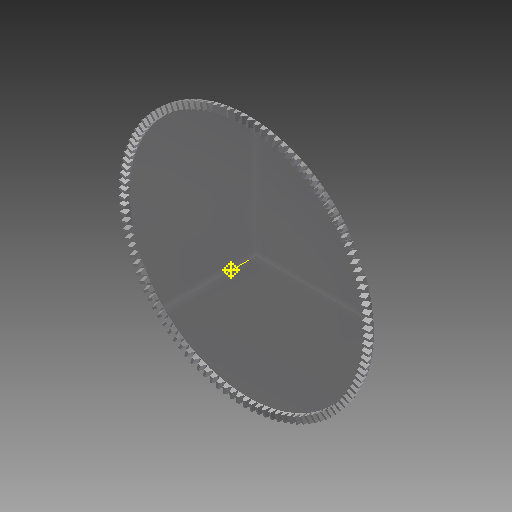
# Autodesk Inventor part: Bevel Gear1
Saved by Autodesk Inventor 2017 (Build 210142000, 142)
## iProperties
Created: 2017-01-10
Part Number: Bevel Gear1
Material: Steel, Mild
Document SubType Name: Modeling
Designer: David Kopala
Categories: <?xml version="1.0" encoding="UTF-16"?> <MemberInstance><Categories><FamilyTemplate><FamilyTemplateParameter ValueType="xs:double" Id="1" ObjectReferenceKey="da_z" ObjectType="kUserParameterObject"/><FamilyTemplateParameter ValueType="xs:double" Id="2" ObjectReferenceKey="da_b" ObjectType="kUserParameterObject"/><FamilyTemplateParameter ValueType="xs:double" Id="3" ObjectReferenceKey="da_beta" ObjectType="kUserParameterObject"/><FamilyTemplateParameter ValueType="xs:double" Id="4" ObjectReferenceKey="da_dae" ObjectType="kUserParameterObject"/><FamilyTemplateParameter ValueType="xs:double" Id="5" ObjectReferenceKey="da_ve" ObjectType="kUserParameterObject"/><FamilyTemplateParameter ValueType="xs:double" Id="6" ObjectReferenceKey="da_omega" ObjectType="kUserParameterObject"/><FamilyTemplateParameter ValueType="xs:string" Id="7" ObjectReferenceKey="EAIAABAAAAAAHwAAAAAAAIAAAAAAAAAA" ObjectType="83914240" SubObjectId="SurfaceGeometry"/></FamilyTemplate><ParamToTemplateMap><ParamToTemplate CategoryParameter="//CategoryParameter[@InternalName='046C89C9-8512-4d59-83FE-43B91F4F132A']" TemplateParameter="1"/><ParamToTemplate CategoryParameter="//CategoryParameter[@InternalName='2552DF32-E462-4b46-AEBF-C6C7768E72AC']" TemplateParameter="2"/><ParamToTemplate CategoryParameter="//CategoryParameter[@InternalName='C9EE641D-15FC-4fae-A226-E94C4372FDD7']" TemplateParameter="3"/><ParamToTemplate><ParamToTemplate CategoryParameter="//CategoryParameter[@InternalName='00B6519A-459B-49c7-AD84-2E56D39A5744']" ConstantValue="0.000000"/></ParamToTemplate><ParamToTemplate><ParamToTemplate CategoryParameter="//CategoryParameter[@InternalName='04B31F0E-C7A6-4894-AA32-9629BEFACF47']" ConstantValue="1.000000"/></ParamToTemplate><ParamToTemplate><ParamToTemplate CategoryParameter="//CategoryParameter[@InternalName='43CBEC2E-7847-49e7-A936-2F7889FCB2D9']" ConstantValue="0.200000"/></ParamToTemplate><ParamToTemplate><ParamToTemplate CategoryParameter="//CategoryParameter[@InternalName='B1EFC894-105D-4ebd-86BF-FA20ED196853']" ConstantValue="0.300000"/></ParamToTemplate><ParamToTemplate><ParamToTemplate CategoryParameter="//CategoryParameter[@InternalName='51175063-3D10-4879-93E8-6246FE8B403D']" ConstantValue="2061532430.657340"/></ParamToTemplate><ParamToTemplate><ParamToTemplate CategoryParameter="//CategoryParameter[@InternalName='A3A52E27-4454-46a9-B0BD-C932399B70AF']" ConstantValue="0.300000"/></ParamToTemplate><ParamToTemplate CategoryParameter="//CategoryParameter[@InternalName='2A200944-5A8C-41ca-B96E-8520D2E510F1']" TemplateParameter="4"/><ParamToTemplate><ParamToTemplate CategoryParameter="//CategoryParameter[@InternalName='1A637F62-92C8-44bc-B81F-10802510B579']" ConstantValue="27.761106"/></ParamToTemplate><ParamToTemplate CategoryParameter="//CategoryParameter[@InternalName='B52DD4BE-6863-48fb-BF58-89EF6F9EC65C']" TemplateParameter="5"/><ParamToTemplate><ParamToTemplate CategoryParameter="//CategoryParameter[@InternalName='3956BFF2-84D2-457d-93C2-9B0613DEBA67']" ConstantValue="1.567608"/></ParamToTemplate><ParamToTemplate CategoryParameter="//CategoryParameter[@InternalName='739CFA02-461B-4bf8-8049-181FCAD8B28F']" TemplateParameter="6"/><ParamToTemplate><ParamToTemplate CategoryParameter="//CategoryParameter[@InternalName='A27E999F-E2CE-4481-8A2A-EBF499C4C3C5']" ConstantValue="0.000000"/></ParamToTemplate><ParamToTemplate><ParamToTemplate CategoryParameter="//CategoryParameter[@InternalName='9E1B4470-B2D3-4ff1-B813-535BB4CDF51A']" ConstantValue="3523220.976809"/></ParamToTemplate><ParamToTemplate><ParamToTemplate CategoryParameter="//CategoryParameter[@InternalName='F8452263-BFF6-458c-9FB1-07C4B99E95CD']" ConstantValue="11397033.805607"/></ParamToTemplate><ParamToTemplate><ParamToTemplate CategoryParameter="//CategoryParameter[@InternalName='3E3BB259-FD49-497f-8171-6EBC954A3479']" ConstantValue="2.000000"/></ParamToTemplate><ParamToTemplate CategoryParameter="//CategoryParameter[@InternalName='27C3BAF2-7550-4e4b-AE2C-0DB134B7D9B7']" TemplateParameter="7"/></ParamToTemplateMap><Category DisplayName="Gear" InternalName="DC85795E-93AB-48d5-8EEE-5A27447B64BD" Mnemonic="Gear"><CategoryParameter DisplayName="z" InternalName="046C89C9-8512-4d59-83FE-43B91F4F132A" Mnemonic="z"/><CategoryParameter DisplayName="b" InternalName="2552DF32-E462-4b46-AEBF-C6C7768E72AC" Mnemonic="b"/><CategoryParameter DisplayName="||b|" InternalName="C9EE641D-15FC-4fae-A226-E94C4372FDD7" Mnemonic="beta"/><CategoryParameter DisplayName="x" InternalName="00B6519A-459B-49c7-AD84-2E56D39A5744" Mnemonic="x"/><CategoryParameter DisplayName="a*" InternalName="04B31F0E-C7A6-4894-AA32-9629BEFACF47" Mnemonic="a"/><CategoryParameter DisplayName="c*" InternalName="43CBEC2E-7847-49e7-A936-2F7889FCB2D9" Mnemonic="c"/><CategoryParameter DisplayName="r|.f|*" InternalName="B1EFC894-105D-4ebd-86BF-FA20ED196853" Mnemonic="rf"/><CategoryParameter DisplayName="E" InternalName="51175063-3D10-4879-93E8-6246FE8B403D" Mnemonic="E"/><CategoryParameter DisplayName="||m|" InternalName="A3A52E27-4454-46a9-B0BD-C932399B70AF" Mnemonic="mi"/><Category DisplayName="BevelGear" InternalName="0C98F69A-0C2B-4791-B2FE-7691BB227E77" Mnemonic="BevelGear"><CategoryParameter DisplayName="d|.ae|" InternalName="2A200944-5A8C-41ca-B96E-8520D2E510F1" Mnemonic="dae"/><CategoryParameter DisplayName="d|.ai|" InternalName="1A637F62-92C8-44bc-B81F-10802510B579" Mnemonic="dai"/><CategoryParameter DisplayName="A|.e|" InternalName="B52DD4BE-6863-48fb-BF58-89EF6F9EC65C" Mnemonic="ve"/><CategoryParameter DisplayName="A|.i|" InternalName="3956BFF2-84D2-457d-93C2-9B0613DEBA67" Mnemonic="vi"/><CategoryParameter DisplayName="||S|" InternalName="739CFA02-461B-4bf8-8049-181FCAD8B28F" Mnemonic="omega"/><CategoryParameter DisplayName="x|.t|" InternalName="A27E999F-E2CE-4481-8A2A-EBF499C4C3C5" Mnemonic="xt"/><CategoryParameter DisplayName="||s||.Flim|" InternalName="9E1B4470-B2D3-4ff1-B813-535BB4CDF51A" Mnemonic="sFlim"/><CategoryParameter DisplayName="||s||.Hlim|" InternalName="F8452263-BFF6-458c-9FB1-07C4B99E95CD" Mnemonic="sHlim"/><CategoryParameter DisplayName="type" InternalName="3E3BB259-FD49-497f-8171-6EBC954A3479" Mnemonic="type"/><CategoryParameter DisplayName="PitchDiameter" InternalName="27C3BAF2-7550-4e4b-AE2C-0DB134B7D9B7" Mnemonic="IDS_PITCHDIAM"/></Category></Category></Categories></MemberInstance>
Mass: 60.9118 g
Surface Area: 34.3074 cm^2
Volume: 7.7496 cm^3
Density: 7.86 g/cm^3
Appearance: Steel
CustomPartVersion: 1
Author: David Kopala
Autodesk Inventor part; units mm, degrees
ref_plane "XZ Plane" through (0, 0, 0) normal (0, 1, 0) x (-1, 0, 0)
ref_plane "Mesh Plane2" through (0, 0, 0) normal (0.9996269, 0.0273148, 0) x (0, 0, 1)
sketch "Teeth Body Sketch" plane through (0, 0, 0) normal (1, 0, 0) x (0, 1, 0)
  line L0 (0, 0) -> (145.6558, -22.0724) construction
  line L1 (145.6558, -22.0724) -> (146.3785, -16.5313)
  line L2 (146.3785, -16.5313) -> (0, 0) construction
  line L3 (146.05, -19.05) -> (0, 0) construction
  line L4 (138.1202, -20.9305) -> (138.8055, -15.6761)
  line L5 (145.6558, -22.0724) -> (138.1202, -20.9305)
  line L6 (146.3785, -16.5313) -> (138.8055, -15.6761)
  line L7 (0, -26.4874) -> (0, 4.4146) projected
  line L8 (0, -19.05) -> (146.3785, -19.05) construction
  dimension "d0" = 292.1
  dimension "d1" = 291.3116
  dimension "d2" = 292.757
  dimension "d3" = 7.62
  dimension "d4" = 16.5313
  constraints: 16 end point, 4 point on line, 3 perpendicular, 2 collinear, 1 horizontal alignment, 1 vertical alignment
  measures "d0" diameter of L3.start L7
  measures "d1" diameter of L0.end L7
  measures "d2" diameter of L1.end L7
  measures "d3" distance between parallel lines of L1 L4
  measures "d4" vertical distance of L1.end L0.start
revolve "Teeth Body" add sketch "Teeth Body Sketch" angle 360 about axis through (0, 0, 0) along (0, 0, 1)
ref_plane "Tooth Plane" through (0, 146.05, -19.05) normal (0, -0.9916004, 0.1293392) x (1, 0, 0)
sketch "Start Sketch" plane through (0, 146.05, -19.05) normal (0, -0.9916004, 0.1293392) x (1, 0, 0)
  line L0 (0, -1379.3559) -> (0, 234.8142) projected
  arc A0 (-0.7258, -3.7185) -> (-3.4846, 4.2111) centre (-367.6879, -126.9464) ccw
  arc A1 (3.4846, 4.2111) -> (0.7258, -3.7185) centre (367.6879, -126.9464) ccw
  line L1 (-0.7258, -3.7185) -> (0.7258, -3.7185)
  arc A2 (3.4846, 4.2111) -> (-3.4846, 4.2111) centre (0, -1129.2015) ccw
  dimension "d7" = 387.0999
  dimension "d8" = 367.6879
  dimension "d9" = 1002.255
  dimension "d57" = 1133.4179
  dimension "d58" = 1125.4829
  constraints: 6 point on circle, 3 centre point, 3 symmetric about line, 2 end point, 1 coincident, 1 perpendicular, 1 other
  measures "d7" radius of A0
  measures "d8" horizontal distance of point (0, -1129.201) A0.centre
  measures "d9" vertical distance of point (0, -1129.201) A0.centre
  measures "d57" radius of A2
  measures "d58" distance from line of A2.centre L1
sketch "End Sketch" plane through (0, 138.217, -18.0283) normal (0, -0.9916004, 0.1293392) x (1, 0, 0)
  line L0 (0, -1306.2352) -> (0, 223.7109) projected
  arc A0 (-0.6876, -2.3936) -> (-3.3012, 5.1186) centre (-348.3356, -119.1357) ccw
  arc A1 (3.3012, 5.1186) -> (0.6876, -2.3936) centre (348.3356, -119.1357) ccw
  line L1 (-0.6876, -2.3936) -> (0.6876, -2.3936)
  arc A2 (3.3012, 5.1186) -> (-3.3012, 5.1186) centre (0, -1068.6394) ccw
  dimension "d12" = 366.7258
  dimension "d15" = 348.3356
  dimension "d16" = 949.5037
  dimension "d59" = 1073.7631
  dimension "d60" = 1066.2458
  constraints: 6 point on circle, 3 centre point, 3 symmetric about line, 2 end point, 1 coincident, 1 other
  measures "d12" radius of A0
  measures "d15" horizontal distance of A0.centre point (0, -1068.639)
  measures "d16" vertical distance of A0.centre point (0, -1068.639)
  measures "d59" radius of A2
  measures "d60" distance from line of A2.centre L1
loft "Loft" cut profiles "Start Sketch", "End Sketch"
pattern_circular "Circular Pattern" count 115 over 360 about axis through (0, 0, 0) along (0, 0, 1) of "Loft"
ref_plane "End Plane" through (0, 138.217, -18.0283) normal (0, -0.9916004, 0.1293392) x (1, 0, 0)
sketch3d "3D Sketch Right"
ref_plane "End Plane Right" through (-2.8237, 138.1881, -18.0283) normal (0.0202578, -0.9913935, 0.1293392) x (0.9997913, 0.0204294, 0)
sketch "End Sketch Right" plane through (-2.8237, 138.1881, -18.0283) normal (0.0202578, -0.9913935, 0.1293392) x (0.9997913, 0.0204294, 0)
  arc A0 (-0.6876, -2.3936) -> (-3.3012, 5.1186) centre (-348.3356, -119.1357) ccw
  line L0 (0, -1308.8574) -> (0, 226.3331) projected
  arc A1 (3.3012, 5.1186) -> (0.6876, -2.3936) centre (348.3356, -119.1357) ccw
  line L1 (-0.6876, -2.3936) -> (0.6876, -2.3936)
  arc A2 (3.3012, 5.1186) -> (-3.3012, 5.1186) centre (0, -1068.6394) ccw
  dimension "d70" = 348.3356
  dimension "d71" = 949.5037
  dimension "d72" = 366.7258
  dimension "d73" = 1066.2458
  dimension "d74" = 1073.7631
  constraints: 6 point on circle, 3 centre point, 3 symmetric about line, 2 end point, 1 coincident, 1 perpendicular, 1 other
  measures "d70" horizontal distance of A2.centre A0.centre
  measures "d71" vertical distance of point (0, -1068.639) A0.centre
  measures "d72" radius of A0
  measures "d73" distance from line of point (0, -1068.639) L1
  measures "d74" radius of A2
feature "Loft Right" [suppressed]
pattern_circular "Circular Pattern Right" [suppressed]
sketch3d "3D Sketch Left"
ref_plane "End Plane Left" through (2.8345, 138.1881, -18.0586) normal (-0.0203346, -0.991364, 0.1295528) x (0.9997897, -0.0205074, 0)
sketch "End Sketch Left" plane through (2.8345, 138.1881, -18.0586) normal (-0.0203346, -0.991364, 0.1295528) x (0.9997897, -0.0205074, 0)
  line L0 (0, -1308.8417) -> (0, 226.3775) projected
  arc A0 (-0.6876, -2.3636) -> (-3.3012, 5.1487) centre (-348.3356, -119.1057) ccw
  arc A1 (3.3012, 5.1487) -> (0.6876, -2.3636) centre (348.3356, -119.1057) ccw
  line L1 (-0.6876, -2.3636) -> (0.6876, -2.3636)
  ellipse E0 centre (0, -15.544) end of major axis (138.8055, -15.544) minor radius 17.9826 projected
  arc A2 (3.3012, 5.1487) -> (-3.3012, 5.1487) centre (0, -1068.6094) ccw
  dimension "d56" = 17.9826
  dimension "d30" = 366.7258
  dimension "d31" = 348.3356
  dimension "d32" = 949.5037
  dimension "d61" = 1073.7631
  dimension "d62" = 1066.2458
  constraints: 6 point on circle, 3 centre point, 3 symmetric about line, 2 end point, 1 coincident, 2 other
  measures "d30" radius of A0
  measures "d31" horizontal distance of point (0, -1068.609) A0.centre
  measures "d32" vertical distance of A0.centre point (0, -1068.609)
  measures "d61" radius of A2
  measures "d62" distance from line of point (0, -1068.609) L1
feature "Loft Left" [suppressed]
pattern_circular "Circular Pattern Left" [suppressed]
sketch "Body Sketch" plane through (0, 0, 0) normal (1, 0, 0) x (0, 1, 0)
  line L0 (0, -22.2993) -> (0, -20.7141) projected
  line L1 (145.6558, -22.0724) -> (138.1202, -20.9305) projected
  line L2 (138.1202, -20.9305) -> (0, -20.9305)
  line L3 (145.6558, -22.0724) -> (0, -22.0724)
  constraints: 4 end point, 2 perpendicular, 2 point on line
revolve "Fix Body" add sketch "Body Sketch" angle 360 about axis through (0, 0, 0) along (0, 0, 1)
sketch "Sketch6" plane through (0, 0, 0) normal (1, 0, 0) x (0, 1, 0)
  line L0 (146.05, -19.05) -> (0, 0) projected
  line L1 (0, -22.86) -> (0, 3.81) projected
surface revolve "Pitch Diameter" sketch "Sketch6" angle 360 about axis through (0, 0, 0) along (0, 0, 1) shown no curves L0
equation "\"d0\" = da_de"
equation "\"d1\" = da_dfe"
equation "\"d2\" = da_dae"
equation "\"d3\" = da_b"
equation "\"d4\" = da_ve"
equation "\"d7\" = fd_rr"
equation "\"d8\" = fd_x"
equation "\"d9\" = fd_y"
equation "\"d57\" = 0.5 * fd_dva + 0.3 * da_he"
equation "\"d58\" = 0.5 * fd_dva - 1.12 * da_he"
equation "\"da_teethtype\" = 0"
equation "\"da_b\" = 7.62"
equation "\"da_de\" = 292.1"
equation "\"da_dae\" = 292.75704"
equation "\"da_dfe\" = 291.31155"
equation "\"da_le\" = 147.28715"
equation "\"da_omega\" = 90deg"
equation "\"da_beta\" = 0"
equation "\"da_delta\" = 82.568592deg"
equation "\"da_alpha\" = 20deg"
equation "\"da_he\" = 5.588"
equation "\"da_ve\" = 16.53133"
equation "\"da_zv\" = 889.135035"
equation "\"fd_loft\" = da_b + 0.05 * da_he"
equation "\"fd_x\" = fd_x1 + fd_x2"
equation "\"fd_y\" = fd_y1 - fd_y2"
equation "\"fd_dd\" = fd_dva - 0.8 * da_he"
equation "\"da_dvw\" = 2258.40299"
equation "\"d11\" = fd_loft"
equation "\"da_dm\" = 284.544"
equation "\"da_x\" = 0"
equation "\"da_m\" = 2.54"
equation "\"d50\" = da_omega"
equation "\"fd_rr\" = 387.099928"
equation "\"fd_dva\" = 2263.482991"
equation "\"fd_x1\" = 1.99491"
equation "\"fd_x2\" = 365.693032"
equation "\"fd_y1\" = 1129.199733"
equation "\"fd_y2\" = 126.944716"
body "Solid1"
body "Srf1"
